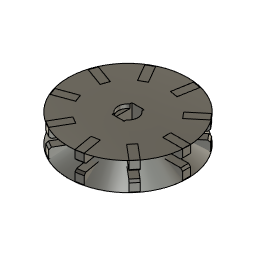
Pulley-40deg (Autodesk Fusion 360 design; units mm, degrees)
Autodesk Fusion 360 part; units mm, degrees
note: some values were not read from the file. Chosen so that the rebuilt part matches the saved one: which bodies a step acts on; which face or edge a step refers to; that a step has no effect; the sign of a taper.
cylinder "CylinderPrimitive1" add diameter 30 height 5 placed x (1, 0, 0) y (0, 1, 0) z (0, 0, 1) at (0, 0, 0) makes body 1
hole "Hole1" at (0, 0, 5) direction (0, 0, -1) diameter 5 end through all bodies 1
delete_face "DeleteFace1" 1 faces at (0.1246, -2.4969, 3.3333) on bodies 1
sketch "Sketch3" plane through (0, 0, 5) normal (0, 0, 1) x (-1, 0, 0)
  circle A0 centre (0, 0) radius 15
  line L0 (-1.5, 2.5) -> (1.5, 2.5)
  line L1 (1.5, 2.5) -> (1.5, -2.5)
  line L2 (1.5, -2.5) -> (-1.5, -2.5)
  line L3 (-1.5, -2.5) -> (-1.5, 2.5)
  line L4 (-1.5, 2.5) -> (1.5, -2.5) construction
  line L5 (1.5, 2.5) -> (-1.5, -2.5) construction
  dimension "d8" = 3
  dimension "d9" = 5
  constraint horizontal L0
  constraint perpendicular L0 L1
  constraint parallel L0 L2
  constraint parallel L1 L3
  constraint coincident L4 A0.centre
  constraint coincident L5 A0.centre
  constraint coincident A0.centre origin
  measures "d8" distance of L1.end L2.end
  measures "d9" distance of L0.end L1.end
extrude "Extrude1" cut sketch "Sketch3" along normal through all and the other way through all contours L0 L1 L2 L3 bodies 1
extrude "Extrude2" add 1 faces at (-6, 0, 5) along direction (0, 0, 1) blind 2 on bodies 1 bodies 1
split "Split1" by plane through (0, 0, 3.5) normal (0, 0, 1) bodies 1 makes body 2 at (-6, 0, 7)
draft "Draft1" angle -60 neutral plane through (0, 0, 3.5) pull (0, 0, 1) 1 faces at (14.9255, 1.4935, 2.3333) on bodies 1
mirror "Mirror1" about plane through (0, 0, 0) normal (0, 0, -1) of bodies 1 makes body 3
combine "Combine1" operation add target body 1 tool bodies 3 result as body 4 in component "Component"
combine "Combine2" [no effect] in component "Component"
sketch "Sketch4" plane through (0, 0, 0) normal (0, 0, 1) x (1, 0, 0)
  line L0 (20, 2) -> (25, 2)
  line L1 (25, 2) -> (25, 0)
  line L2 (25, 0) -> (20, 0)
  line L3 (20, 0) -> (20, 2)
  dimension "d17" = 5
  constraint horizontal L0
  constraint vertical L1
  constraint horizontal L2
  constraint vertical L3
  measures "d17" distance of L0.start L0.end
extrude "Extrude3" add sketch "Sketch4" along normal blind 2 separate body makes body 5
copy_body "CopyPasteBodies2" bodies 5 makes body 6
move_body "Move3" bodies 6 to x (1, 0, 0) y (0, 1, 0) z (0, 0, 1) at (0, 0, 5)
move_body "Move4" bodies 5 to x (1, 0, 0) y (0, 1, 0) z (0, 0, 1) at (-10.1448, -1.1172, -3.4596)
move_body "Move5" bodies 6 to x (1, 0, 0) y (0, 1, 0) z (0, 0, 1) at (-9.1389, -1.0916, -3.8351)
move_body "Move6" bodies 6 to x (1, 0, 0) y (0, 1, 0) z (0, 0, 1) at (-1.1069, -0.1825, 0.3653)
move_body "Move7" bodies 6 to x (1, 0, 0) y (0, 1, 0) z (0, 0, 1) at (-0.0027, 0.1354, 0.0193)
move_body "Move8" bodies 6 to x (1, 0, 0) y (0, 1, 0) z (0, 0, 1) at (0.0121, 0.0175, -0.0574)
move_body "Move9" bodies 6 to x (1, 0, 0) y (0, 1, 0) z (0, 0, 1) at (0.0769, 0.0087, 0.0194)
ref_plane "WorkPlane3" through (0, 0, 12.125) normal (0, 1, 0) x (0, 0, 1)
ref_plane "WorkPlane5" through (0, 0, 0) normal (-1, 0, 0) x (0, 0, 1)
ref_plane "WorkPlane6" through (0, 0, 0) normal (-0.707107, 0.707107, 0) x (0, 0, 1)
ref_plane "WorkPlane7" through (0, 0, 0) normal (0.707107, 0.707107, 0) x (0, 0, 1)
move_body "Move10" bodies 6 to x (1, 0, 0) y (0, 1, 0) z (0, 0, 1) at (0.027, -0.0024, -0.0548)
sketch "Sketch5" plane through (0, 0, -1.4596) normal (0, 0, 1) x (-1, 0, 0)
  line L0 (-9.8552, 1.1172) -> (-14.8552, 1.1172)
  line L1 (-14.8552, 1.1172) -> (-14.8552, -0.8828)
  line L2 (-14.8552, -0.8828) -> (-9.8552, -0.8828)
  line L3 (-9.8552, -0.8828) -> (-9.8552, 1.1172)
  line L4 (-11.2943, -9.7142) -> (-9.88, -11.1284)
  line L5 (-1.1172, -14.8552) -> (0.8828, -14.8552)
  line L6 (9.7142, -11.2943) -> (11.1284, -9.88)
  line L7 (14.8552, -1.1172) -> (14.8552, 0.8828)
  line L8 (11.2943, 9.7142) -> (9.88, 11.1284)
  line L9 (1.1172, 14.8552) -> (-0.8828, 14.8552)
  line L10 (-9.7142, 11.2943) -> (-11.1284, 9.88)
  line L11 (-26.7698, -6.9008) -> (-31.7698, -6.9008)
  line L12 (-31.7698, -6.9008) -> (-31.7698, -4.9008)
  line L13 (-31.7698, -4.9008) -> (-26.7698, -4.9008)
  line L14 (-26.7698, -4.9008) -> (-26.7698, -6.9008)
  dimension "d26" = 360
  dimension "d27" = 5
  dimension "d28" = 2
  constraint horizontal L11
  constraint vertical L12
  constraint horizontal L13
  constraint vertical L14
  measures "d27" distance of L11.start L11.end
  measures "d28" distance of L11.start L13.end
extrude "Extrude7" add 1 faces at (11.5342, 0.2184, 1.4566) along direction (0, 0, -1) blind 0.5 on bodies 6 bodies 6
extrude "Extrude8" add 1 faces at (11.5219, 0.2161, -1.4596) along direction (0, 0, 1) blind 0.5 on bodies 5 bodies 5
chamfer "Chamfer1" distance 0.5 angle 45 1 edges at (14.8552, -0.1172, -0.9596) on bodies 5
chamfer "Chamfer2" distance 0.5 angle 45 1 edges at (14.8675, -0.115, 0.9566) on bodies 6
copy_body "CopyPasteBodies16" bodies 6 makes body 7
move_body "Move37" bodies 7 to x (0.766044, 0.642788, 0) y (-0.642788, 0.766044, 0) z (0, 0, 1) at (0, 0, 0)
copy_body "CopyPasteBodies17" bodies 7 makes body 8
move_body "Move38" bodies 8 to x (0.766044, 0.642788, 0) y (-0.642788, 0.766044, 0) z (0, 0, 1) at (0, 0, 0)
copy_body "CopyPasteBodies18" bodies 8 makes body 9
move_body "Move39" bodies 9 to x (0.766044, 0.642788, 0) y (-0.642788, 0.766044, 0) z (0, 0, 1) at (0, 0, 0)
copy_body "CopyPasteBodies19" bodies 9 makes body 10
move_body "Move40" bodies 10 to x (0.766044, 0.642788, 0) y (-0.642788, 0.766044, 0) z (0, 0, 1) at (0, 0, 0)
copy_body "CopyPasteBodies20" bodies 10 makes body 11
move_body "Move41" bodies 11 to x (0.766044, 0.642788, 0) y (-0.642788, 0.766044, 0) z (0, 0, 1) at (0, 0, 0)
copy_body "CopyPasteBodies21" bodies 11 makes body 12
move_body "Move42" bodies 12 to x (0.766044, 0.642788, 0) y (-0.642788, 0.766044, 0) z (0, 0, 1) at (0, 0, 0)
copy_body "CopyPasteBodies22" bodies 12 makes body 13
move_body "Move43" bodies 13 to x (0.766044, 0.642788, 0) y (-0.642788, 0.766044, 0) z (0, 0, 1) at (0, 0, 0)
copy_body "CopyPasteBodies23" bodies 13 makes body 14
move_body "Move44" bodies 14 to x (0.766044, 0.642788, 0) y (-0.642788, 0.766044, 0) z (0, 0, 1) at (0, 0, 0)
copy_body "CopyPasteBodies24" bodies 5 makes body 15
move_body "Move45" bodies 15 to x (0.766044, 0.642788, 0) y (-0.642788, 0.766044, 0) z (0, 0, 1) at (0, 0, 0)
copy_body "CopyPasteBodies25" bodies 15 makes body 16
move_body "Move46" bodies 16 to x (0.766044, 0.642788, 0) y (-0.642788, 0.766044, 0) z (0, 0, 1) at (0, 0, 0)
copy_body "CopyPasteBodies26" bodies 16 makes body 17
move_body "Move47" bodies 17 to x (0.766044, 0.642788, 0) y (-0.642788, 0.766044, 0) z (0, 0, 1) at (0, 0, 0)
copy_body "CopyPasteBodies27" bodies 17 makes body 18
move_body "Move48" bodies 18 to x (0.766044, 0.642788, 0) y (-0.642788, 0.766044, 0) z (0, 0, 1) at (0, 0, 0)
copy_body "CopyPasteBodies28" bodies 18 makes body 19
move_body "Move49" bodies 19 to x (0.766044, 0.642788, 0) y (-0.642788, 0.766044, 0) z (0, 0, 1) at (0, 0, 0)
copy_body "CopyPasteBodies29" bodies 19 makes body 20
move_body "Move50" bodies 20 to x (0.766044, 0.642788, 0) y (-0.642788, 0.766044, 0) z (0, 0, 1) at (0, 0, 0)
copy_body "CopyPasteBodies30" bodies 20 makes body 21
move_body "Move51" bodies 21 to x (0.766044, 0.642788, 0) y (-0.642788, 0.766044, 0) z (0, 0, 1) at (0, 0, 0)
copy_body "CopyPasteBodies31" bodies 21 makes body 22
move_body "Move52" bodies 22 to x (0.766044, 0.642788, 0) y (-0.642788, 0.766044, 0) z (0, 0, 1) at (0, 0, 0)
hole "Hole1'" at (0, 0, 3.5) direction (0, 0, -1) diameter 5 depth 1 tip angle 180 bodies 4 in component "Component"
component "Component" placed x (1, 0, 0) y (0, 1, 0) z (0, 0, 1) at (0, 0, 0)
hidden bodies 2
named bodies: "Master bund", "Master top", "Master top (1)", "Master top (1) (1)", "Master top (1) (1) (1)", "Master top (1) (1) (1) (1)", "Master top (1) (1) (1) (1) (1)", "Master top (1) (1) (1) (1) (1) (1)", "Master top (1) (1) (1) (1) (1) (1) (1)", "Master top (1) (1) (1) (1) (1) (1) (1) (1)", "Master bund (1)", "Master bund (1) (1)", "Master bund (1) (1) (1)", "Master bund (1) (1) (1) (1)", "Master bund (1) (1) (1) (1) (1)", "Master bund (1) (1) (1) (1) (1) (1)", "Master bund (1) (1) (1) (1) (1) (1) (1)", "Master bund (1) (1) (1) (1) (1) (1) (1) (1)"
